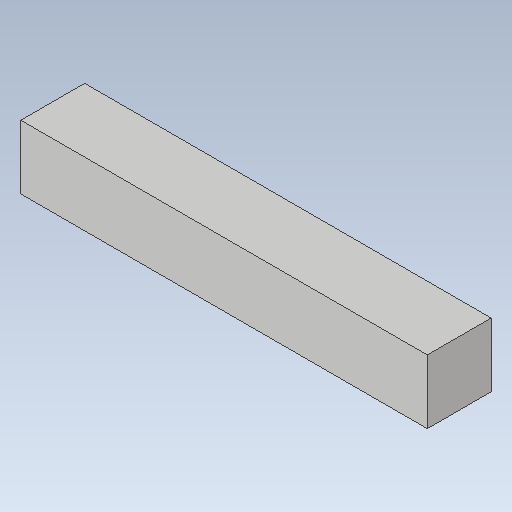
# Autodesk Inventor part: 零件1
Saved by Autodesk Inventor 2020 (Build 240168000, 168)
## iProperties
Created: 2021-06-23
Part Number: 零件1
Material: 常规
Document SubType Name: Modeling
Designer: chenpeizhi66
Density: 1 g/cm^3
Appearance: 默认
Author: chenpeizhi66
Autodesk Inventor part; units mm, degrees
ref_plane "YZ Plane" through (0, 0, 0) normal (1, 0, 0) x (0, 1, 0)
ref_plane "XZ Plane" through (0, 0, 0) normal (0, 1, 0) x (-1, 0, 0)
ref_plane "XY Plane" through (0, 0, 0) normal (0, 0, 1) x (1, 0, 0)
sketch "草图1" plane through (0, 0, 0) normal (0, 0, 1) x (1, 0, 0)
  line L0 (70, 11) -> (70, -11) projected
  line L1 (-70, 11) -> (70, 11) projected
  line L2 (-70, -11) -> (-70, 11) projected
  line L3 (70, -11) -> (-70, -11) projected
  line L4 (70, -11) -> (-70, -11)
  line L5 (-70, -11) -> (-70, 11)
  line L6 (-70, 11) -> (70, 11)
  line L7 (70, 11) -> (70, -11)
  point P0 (0, 0)
  constraints: 8 end point, 2 parallel, 1 horizontal, 1 perpendicular
extrude "拉伸1" add sketch "草图1" along normal blind 22
